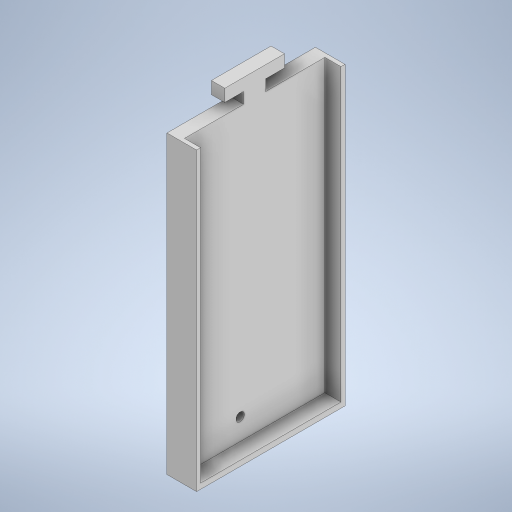
# Autodesk Inventor part: pumpholderfinal
Saved by Autodesk Inventor 2023 (Build 270158000, 158)
## iProperties
Created: 2025-08-30
Part Number: pumpholderfinal
Material: Generic
Document SubType Name: Modeling
Designer: ptato_qo49uko
Density: 1 g/cm^3
Appearance: Default
Author: ptato_qo49uko
Autodesk Inventor part; units mm, degrees
ref_plane "YZ Plane" through (0, 0, 0) normal (1, 0, 0) x (0, 1, 0)
ref_plane "XZ Plane" through (0, 0, 0) normal (0, 1, 0) x (-1, 0, 0)
ref_plane "XY Plane" through (0, 0, 0) normal (0, 0, 1) x (1, 0, 0)
sketch "Sketch1" plane through (0, 0, 0) normal (1, 0, 0) x (0, 1, 0)
  line L0 (62.3549, 27.169) -> (-47.6451, 27.169)
  line L1 (-47.6451, 27.169) -> (-47.6451, -28.031)
  line L2 (-47.6451, -28.031) -> (62.3549, -28.031)
  line L3 (62.3549, -28.031) -> (62.3549, 27.169)
  point P0 (0, 0)
  dimension "d0" = 110
  dimension "d1" = 55.2
  constraints: 8 end point, 2 parallel, 1 horizontal, 1 perpendicular
  measures "d0" distance of L2.end L1.end
  measures "d1" distance of L1.end L0.end
extrude "Extrusion1" add sketch "Sketch1" along normal blind 5
sketch "Sketch3" plane through (5, 0, 0) normal (1, 0, 0) x (0, 0, -1)
  line L0 (-27.169, -47.6451) -> (28.031, -47.6451) projected
  line L1 (28.031, -47.6451) -> (-4.969, -47.6451)
  line L2 (-4.969, -47.6451) -> (-4.969, -37.6451)
  point P0 (0, 0)
  dimension "d12" = 33
  dimension "d13" = 10
  constraints: 4 end point, 1 point on line, 1 vertical
  measures "d12" distance of L0.end L1.end
  measures "d13" distance of L1.end L2.end
hole "Hole2" at (5, -37.6451, 4.969) direction (-1, 0, 0) diameter 3.2 end through all
sketch "Sketch13" plane through (5, 0, 0) normal (1, 0, 0) x (0, 0, -1)
  line L0 (-27.169, -47.6451) -> (28.031, -47.6451) projected
  line L1 (28.031, 62.3549) -> (-27.169, 62.3549) projected
  line L2 (28.031, -47.6451) -> (26.531, -47.6451)
  line L3 (26.531, -47.6451) -> (26.531, 62.3549)
  line L4 (26.531, 62.3549) -> (28.031, 62.3549)
  line L5 (28.031, 62.3549) -> (28.031, -47.6451)
  line L6 (-27.169, 62.3549) -> (-27.169, -47.6451) projected
  line L7 (28.031, 62.3549) -> (-27.169, 62.3549) projected
  line L8 (-27.169, -47.6451) -> (-25.669, -47.6451)
  line L9 (-25.669, -47.6451) -> (-25.669, 62.3549)
  line L10 (-25.669, 62.3549) -> (-27.169, 62.3549)
  line L11 (-27.169, 62.3549) -> (-27.169, -47.6451)
  line L12 (28.031, -47.6451) -> (-27.169, -47.6451)
  line L13 (-27.169, -47.6451) -> (-27.169, -45.6451)
  line L14 (-27.169, -45.6451) -> (28.031, -45.6451)
  line L15 (28.031, -45.6451) -> (28.031, -47.6451)
  point P0 (0, 0)
  point P1 (10.031, 62.3549)
  point P2 (-5.969, 62.3549)
  point P3 (26.531, -45.6451)
  point P4 (-25.669, -45.6451)
  point P5 (18.031, 62.3549)
  dimension "d42" = 1.5
  dimension "d43" = 1.5
  dimension "d44" = 2
  constraints: 24 end point, 6 parallel, 3 horizontal, 3 perpendicular, 3 point on line
  measures "d42" distance of L3.end L4.end
  measures "d43" distance of L10.end L9.end
  measures "d44" distance of L12.end L13.end
extrude "Extrusion7" add sketch "Sketch13" along normal blind 6 contours L6 L14 L9 L0 | L9 L14 L3 L0 | L6 L1 L9 L14 | L3 L14 L5 L0 | L3 L1 L5 L14
sketch "Sketch14" plane through (0, 62.3549, 27.169) normal (0, 1, 0) x (1, 0, 0)
  line L0 (5, 1.5) -> (5, 53.7) projected
  line L1 (5, 53.7) -> (5, 38.7)
  line L2 (5, 1.5) -> (5, 16.5)
  line L3 (5, 38.7) -> (0, 38.7)
  line L4 (5, 21.7) -> (5, 38.7)
  line L5 (0, 55.2) -> (0, 0) projected
  line L6 (5, 38.7) -> (0, 38.7)
  line L7 (0, 38.7) -> (0, 16.5)
  line L8 (0, 16.5) -> (5, 16.5)
  line L9 (5, 16.5) -> (5, 38.7)
  point P0 (0, 27.169)
  dimension "d47" = 15
  dimension "d48" = 15
  constraints: 16 end point, 3 point on line, 2 horizontal, 2 parallel, 1 perpendicular
  measures "d47" distance of L0.end L1.end
  measures "d48" distance of L0.start L2.end
extrude "Extrusion8" add sketch "Sketch14" along normal blind 8.65
sketch "Sketch15" plane through (5, 0, 0) normal (1, 0, 0) x (0, 0, -1)
  line L0 (28.031, 62.3549) -> (11.531, 62.3549) projected
  line L1 (11.531, 62.3549) -> (4.531, 62.3549)
  line L2 (4.531, 62.3549) -> (4.531, 66.4495)
  line L3 (4.531, 66.4495) -> (11.531, 66.4495)
  line L4 (11.531, 66.4495) -> (11.531, 62.3549)
  line L5 (-10.669, 62.3549) -> (-25.669, 62.3549) projected
  line L6 (-10.669, 62.3549) -> (-3.669, 62.3549)
  line L7 (-3.669, 62.3549) -> (-3.669, 66.4495)
  line L8 (-3.669, 66.4495) -> (-10.669, 66.4495)
  line L9 (-10.669, 66.4495) -> (-10.669, 62.3549)
  point P0 (0, 0)
  dimension "d51" = 7
  dimension "d52" = 7
  dimension "d55" = 4.0946
  constraints: 16 end point, 4 parallel, 2 horizontal, 2 perpendicular, 1 point on line
  measures "d51" distance of L2.end L3.end
  measures "d52" distance of L8.end L7.end
  measures "d55" distance of L6.end L7.end
extrude "Extrusion9" cut sketch "Sketch15" against normal blind 8.65
body "Solid1"
